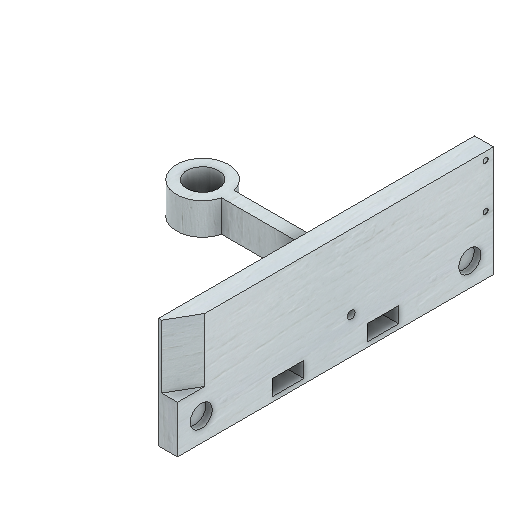
# Autodesk Inventor part: Стенка конвейера
Saved by Autodesk Inventor 2022 (Build 260153000, 153)
## iProperties
Created: 2023-02-18
Part Number: Стенка конвейера
Material: Типовые
Document SubType Name: Modeling
Designer: Глеб
Density: 1 g/cm^3
Appearance: Дерево — окрашенное — белое
Author: Глеб
Autodesk Inventor part; units mm, degrees
ref_plane "YZ Plane" through (0, 0, 0) normal (1, 0, 0) x (0, 1, 0)
ref_plane "XZ Plane" through (0, 0, 0) normal (0, 1, 0) x (-1, 0, 0)
ref_plane "XY Plane" through (0, 0, 0) normal (0, 0, 1) x (1, 0, 0)
sketch "Эскиз1" plane through (0, 0, 0) normal (1, 0, 0) x (0, 1, 0)
  line L0 (0, 100) -> (0, -100)
  line L1 (0, -100) -> (30, -100)
  line L2 (30, -100) -> (30, 100)
  line L3 (30, 100) -> (0, 100)
  line L4 (-14, 0) -> (84, 0) construction
  line L5 (0, -140) -> (0, 140) construction
  line L6 (30, -100) -> (70, -100)
  line L7 (70, -100) -> (70, 100)
  line L8 (70, 100) -> (30, 100)
  line L9 (30, 100) -> (30, -100)
  point P0 (0, 0)
  point P1 (30, 100)
  dimension "d0" = 200
  dimension "d1" = 30
  dimension "d2" = 200
  dimension "d3" = 40
  constraints: 16 end point, 4 parallel, 2 perpendicular, 1 midpoint, 1 point on line, 1 vertical, 1 other
  measures "d0" distance between parallel lines of L3 L1
  measures "d1" distance between parallel lines of L0 L2
  measures "d2" distance of L6.end L7.end
  measures "d3" distance between parallel lines of L2 L7
extrude "Выдавливание1" add sketch "Эскиз1" along normal mid plane 12
sketch "Эскиз2" plane through (6, 0, 0) normal (1, 0, 0) x (0, 0, -1)
  line L0 (-20, 13) -> (-40, 13)
  line L1 (-100, 0) -> (100, 0) construction
  line L2 (100, 0) -> (100, 70) projected
  line L3 (-40, 13) -> (-20, 13)
  line L4 (-20, 13) -> (-20, 3)
  line L5 (-20, 3) -> (-40, 3)
  line L6 (-40, 3) -> (-40, 13)
  line L7 (20, 13) -> (40, 13)
  line L8 (40, 13) -> (40, 3)
  line L9 (40, 3) -> (20, 3)
  line L10 (20, 3) -> (20, 13)
  point P0 (0, 0)
  point P1 (-85, 0)
  point P2 (57.0517, 0.6179)
  dimension "d26" = 10
  dimension "d27" = 20
  dimension "d28" = 3
  dimension "d29" = 20
  dimension "d31" = 20
  dimension "d34" = 3
  dimension "d35" = 10
  dimension "d36" = 20
  constraints: 18 end point, 4 parallel, 2 horizontal, 2 perpendicular
  measures "d26" distance between parallel lines of L0 L5
  measures "d27" distance between parallel lines of L4 L6
  measures "d28" distance between parallel lines of L1 L5
  measures "d29" distance from line of point (0, 0) L4
  measures "d31" distance between parallel lines of L8 L10
  measures "d34" distance between parallel lines of L1 L9
  measures "d35" distance of L9.end L7.start
  measures "d36" distance from line of point (0, 0) L10
extrude "Выдавливание2" cut sketch "Эскиз2" against normal blind 12
sketch "Эскиз3" plane through (6, 0, 0) normal (1, 0, 0) x (0, 0, -1)
  line L0 (100, 0) -> (100, 70) projected
  line L1 (100, 0) -> (-100, 0) projected
  line L2 (-100, 0) -> (-100, 70) projected
  point P0 (0, 0)
  point P1 (-85, 15)
  point P2 (-85, 0)
  point P3 (-85, 15)
  point P4 (85, 15)
  point P5 (-100, 15)
  dimension "d17" = 15
  dimension "d53" = 15
  dimension "d54" = 15
  constraints: 1 coincident
  measures "d17" distance from line of L0 point (85, 15)
  measures "d53" distance from line of L1 point (85, 15)
  measures "d54" distance from line of L2 point (-85, 15)
hole "Отверстие1" at (6, 15, -85) at (6, 15, 85) direction (-1, 0, 0) diameter 14 depth 4.1
sketch "Эскиз4" plane through (6, 0, 0) normal (1, 0, 0) x (0, 0, -1)
  line L0 (100, 70) -> (-100, 70) projected
  line L1 (-100, 70) -> (-100, 0) projected
  line L2 (90, 30) -> (-85, 30) projected
  line L3 (100, 0) -> (100, 70) projected
  line L4 (100, 0) -> (-100, 0) projected
  point P0 (0, 0)
  point P1 (95, 65)
  point P2 (95, 37)
  point P3 (-100, 15)
  point P4 (-85, 0)
  dimension "d37" = 5
  dimension "d40" = 5
  dimension "d51" = 5
  dimension "d52" = 37
  constraints: 1 other
  measures "d37" distance from line of L0 point (95, 65)
  measures "d40" distance from line of L3 point (95, 37)
  measures "d51" distance from line of L3 point (95, 65)
  measures "d52" distance from line of L4 point (95, 37)
hole "Отверстие2" at (6, 65, -95) at (6, 37, -95) direction (-1, 0, 0) diameter 3 depth 70
chamfer "Фаска1" distance 0.2 angle 45 4 edges at (6, 37, -93.5) (6, 65, -93.5) (-6, 37, -93.5) (-6, 65, -93.5)
sketch "Эскиз5" plane through (-6, 70, 100) normal (0, 1, 0) x (1, 0, 0)
  line L0 (12, 0) -> (0, 0) projected
  line L1 (2, 0) -> (12, 17.3205)
  line L2 (12, 200) -> (12, 0) projected
  line L3 (12, 0) -> (2, 0)
  line L4 (12, 15) -> (12, 0) projected
  line L5 (12, 0) -> (12, 17.3205)
  point P0 (6, 100)
  dimension "d60" = 30
  dimension "d61" = 10
  constraints: 6 end point, 2 point on line, 1 horizontal, 1 vertical
  measures "d60" angle of L2 L1
  measures "d61" distance of L0.start L1.start
extrude "Выдавливание3" cut sketch "Эскиз5" against normal blind 40
sketch "Эскиз6" plane through (-6, 0, 0) normal (-1, 0, 0) x (0, 0, 1)
  line L0 (-40, 13) -> (-20, 13) projected
  point P0 (0, 0)
  point P1 (-10, 23)
  dimension "d62" = 10
  dimension "d63" = 10
  measures "d62" distance from line of L0 point (-10, 23)
  measures "d63" horizontal distance of point (0, 0) point (-10, 23)
hole "Отверстие3" at (-6, 23, -10) direction (1, 0, 0) diameter 5 depth 60
sketch "Эскиз7" plane through (-6, 0, 0) normal (-1, 0, 0) x (0, 0, 1)
  line L0 (-4, 60) -> (4, 60)
  line L1 (4, 60) -> (4, 40)
  line L2 (4, 40) -> (-4, 40)
  line L3 (-4, 40) -> (-4, 60)
  line L4 (0, 0) -> (0, 6.9143) construction
  line L5 (-100, 0) -> (100, 0) projected
  dimension "d71" = 8
  dimension "d72" = 20
  dimension "d73" = 40
  constraints: 10 end point, 2 parallel, 1 horizontal, 1 perpendicular, 1 vertical, 1 other
  measures "d71" distance between parallel lines of L1 L3
  measures "d72" distance between parallel lines of L2 L0
  measures "d73" distance between parallel lines of L5 L2
extrude "Выдавливание4" add sketch "Эскиз7" along normal blind 61
sketch "Эскиз10" plane through (-6, 40, -4) normal (0, -1, 0) x (1, 0, 0)
  line L0 (-104, -147.0883) -> (-50, -147.0883) projected
  line L1 (-50, 252.9117) -> (-50, -147.0883) construction
  circle A0 centre (-72.15, -8.6973) radius 16.5 construction
  circle A1 centre (-72.15, -8.6973) radius 10 construction
  circle A2 centre (-72.15, -8.6973) radius 10 construction
  circle A3 centre (-72.15, -8.6973) radius 11 construction
  circle A4 centre (-72.15, 4) radius 16.5
  circle A5 centre (-72.15, 4) radius 11
  circle A6 centre (-72.15, 4) radius 10
  line L2 (-50, 252.9117) -> (-104, 252.9117) projected
  line L3 (-104, -147.0883) -> (-104, 252.9117) projected
  point P0 (6, 4)
  point P1 (-100, 252.9117)
  dimension "d86" = 33
  dimension "d87" = 22
  dimension "d88" = 20
  constraints: 3 centre point, 2 coincident
  measures "d86" diameter of A4
  measures "d87" diameter of A5
  measures "d88" diameter of A6
extrude "Выдавливание6" add sketch "Эскиз10" against normal blind 20 contours A4 | A5
equation "\"d40\" = d37"
